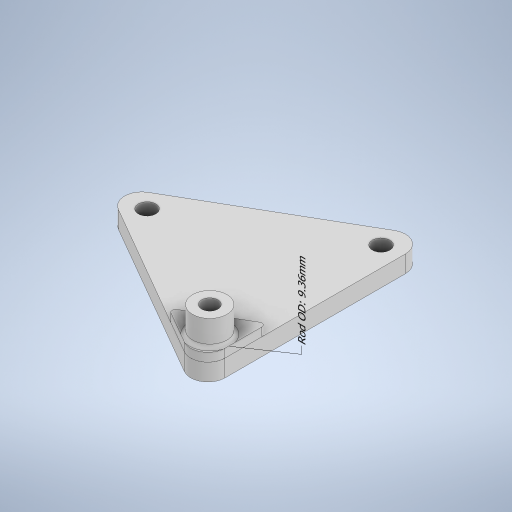
# Autodesk Inventor part: base
Saved by Autodesk Inventor 2023 (Build 270158000, 158)
## iProperties
Created: 2022-11-10
Part Number: base
Material: Generic
Document SubType Name: Modeling
Designer: eahil
Density: 1 g/cm^3
Appearance: Default
Author: eahil
Autodesk Inventor part; units mm, degrees
ref_plane "YZ Plane" through (0, 0, 0) normal (1, 0, 0) x (0, 1, 0)
ref_plane "XZ Plane" through (0, 0, 0) normal (0, 1, 0) x (-1, 0, 0)
ref_plane "XY Plane" through (0, 0, 0) normal (0, 0, 1) x (1, 0, 0)
sketch "Sketch1" plane through (0, 0, 0) normal (0, 1, 0) x (-1, 0, 0)
  circle A0 centre (0, 0) radius 5.127
  circle A1 centre (0, -100) radius 5.127
  circle A2 centre (86.6025, -50) radius 5.127
  line L0 (0, -100) -> (0, 0)
  line L1 (0, 0) -> (86.6025, -50)
  line L2 (86.6025, -50) -> (0, -100)
  line L3 (-11.547, -102.6795) -> (-11.547, 2.6795)
  line L4 (3.453, 11.3397) -> (94.6966, -41.3397)
  line L5 (94.6966, -58.6603) -> (3.453, -111.3397)
  arc A3 (94.6966, -58.6603) -> (94.6966, -41.3397) centre (89.6966, -50) ccw
  arc A4 (-11.547, -102.6795) -> (3.453, -111.3397) centre (-1.547, -102.6795) ccw
  arc A5 (3.453, 11.3397) -> (-11.547, 2.6795) centre (-1.547, 2.6795) ccw
  point P0 (28.8675, -50)
  point P1 (28.8675, -50)
  point P2 (-11.547, -120)
  point P3 (-11.547, 20)
  point P4 (109.6966, -50)
  dimension "d0" = 10.254
  dimension "d1" = 100
  dimension "d2" = 140
  dimension "d3" = 10
  constraints: 12 end point, 6 centre point, 6 point on circle, 6 point on line, 6 tangent, 5 coincident, 4 equal radius, 1 parallel, 1 vertical alignment, 14 other
  measures "d0" diameter of A0
  measures "d1" distance of A1.centre point (0, 0)
  measures "d2" distance of point (109.697, -50) point (-11.547, -120)
  measures "d3" radius of A3
extrude "Extrusion1" add sketch "Sketch1" along normal blind 10 contours A0 L1 A2 L2 A1 L0 | L3 A5 L4 A3 L5 A4
sketch "Sketch2" plane through (0, 10, 0) normal (0, 1, 0) x (1, 0, 0)
  arc A0 (-3.453, -11.3397) -> (11.547, -2.6795) centre (1.547, -2.6795) ccw projected
  line L0 (-94.6966, 41.3397) -> (-3.453, -11.3397) projected
  line L1 (-3.453, -11.3397) -> (-22.1036, -0.5718)
  line L2 (-22.1036, 2.8923) -> (8.547, 20.5885)
  line L3 (11.547, -2.6795) -> (11.547, 102.6795) projected
  line L4 (11.547, -2.6795) -> (11.547, 18.8564)
  arc A1 (-22.1036, 2.8923) -> (-22.1036, -0.5718) centre (-21.1036, 1.1603) ccw
  arc A2 (11.547, 18.8564) -> (8.547, 20.5885) centre (9.547, 18.8564) ccw
  circle A3 centre (0, 0) radius 4.7435
  point P0 (-25.1036, 1.1603)
  point P1 (11.547, 22.3205)
  point P2 (-22.1036, -0.5718)
  dimension "d6" = 25
  dimension "d7" = 25
  dimension "d8" = 2
  dimension "d11" = 9.487
  constraints: 6 end point, 6 point on line, 4 point on circle, 4 tangent, 3 centre point, 1 coincident, 1 collinear, 1 equal radius
  measures "d6" distance of L0.end point (-25.104, 1.16)
  measures "d7" distance of L3.start point (11.547, 22.321)
  measures "d8" radius of A1
  measures "d11" diameter of A3
extrude "Extrusion2" add sketch "Sketch2" along normal blind 5 separate body
sketch "Sketch3" plane through (0, 15, 0) normal (0, 1, 0) x (1, 0, 0)
  circle A0 centre (0, 0) radius 10
  circle A1 centre (0, 0) radius 4.7435
  dimension "d14" = 20
  constraints: 2 centre point, 2 coincident
  measures "d14" diameter of A0
extrude "Extrusion3" add sketch "Sketch3" along normal blind 15 bodies 2
fillet "Fillet1" radius 2 1 edges at (-10, 15, 0)
body "Solid1"
